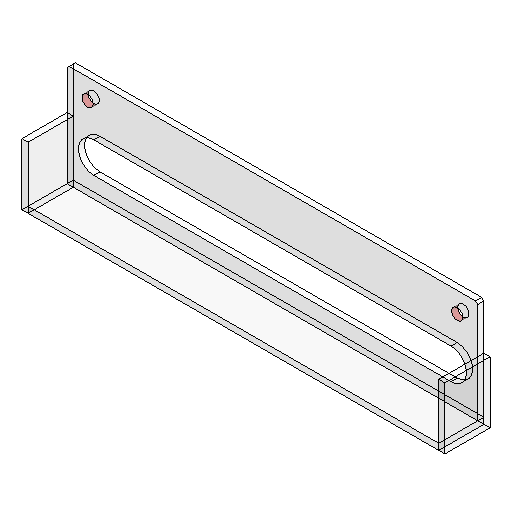
# Autodesk Inventor part: TL20240901-10320CV-027
Saved by Autodesk Inventor 2022.5 (Build 265521000, 521)
## iProperties
Category: FOLLOWER UNIT ASSY
Company: 현대 트랜시스
RuleStatus: InUse
Part Number: TL20240901-10320CV-027
Project: MEa-PJT 2LINE
Checked By: 김형민
Engr Approved By: 김형민
User Status: 2 x6
Material: PC
Description: 0
Document SubType Name: Modeling
Mfg Approved By: 호상태
Designer: USER106
Stock Number: 027
Density: 0.357273 g/cm^3
Appearance: Transparency
Detail Description: Processed products
Title: COVER
Subject: MEa차종 시트조립2라인
Author: USER106
Revision Number: A
Autodesk Inventor part; units mm, degrees
ref_plane "YZ Plane" through (0, 0, 0) normal (1, 0, 0) x (0, 1, 0)
ref_plane "XZ Plane" through (0, 0, 0) normal (0, 1, 0) x (-1, 0, 0)
ref_plane "XY Plane" through (0, 0, 0) normal (0, 0, 1) x (1, 0, 0)
sketch "Sketch2" plane through (0, 0, 0) normal (0, 1, 0) x (-1, 0, 0)
  line L0 (-100, -25) -> (100, -25)
  line L1 (100, -25) -> (100, 25)
  line L2 (100, 25) -> (-100, 25)
  line L3 (-100, 25) -> (-100, -25)
  line L4 (-100, -25) -> (100, 25) construction
  line L5 (100, -25) -> (-100, 25) construction
  point P0 (0, 0)
  dimension "d1" = 200
  dimension "d2" = 50
  constraints: 12 end point, 2 midpoint, 2 parallel, 1 horizontal, 1 perpendicular
  measures "d1" distance of L1.end L2.end
  measures "d2" distance of L0.end L1.end
extrude "Extrusion1" add sketch "Sketch2" along normal mid plane 3
sketch "Sketch3" plane through (100, -1.5, -25) normal (1, 0, 0) x (0, 0, -1)
  line L0 (-27, 3) -> (3, 3)
  line L1 (3, 3) -> (3, -19)
  line L2 (3, -19) -> (-27, -19)
  line L3 (-27, -19) -> (-27, 3)
  line L4 (0, 0) -> (0, 3) projected
  line L5 (-50, 3) -> (0, 3) projected
  point P0 (-25, 1.5)
  dimension "d13" = 3
  dimension "d14" = 22
  dimension "d15" = 30
  constraints: 8 end point, 2 parallel, 1 horizontal, 1 perpendicular, 1 point on line
  measures "d13" distance between parallel lines of L4 L1
  measures "d14" distance of L0.end L1.end
  measures "d15" distance of L0.start L0.end
extrude "Extrusion2" add sketch "Sketch3" along normal blind 3 separate body
extrude "Extrusion3" add sketch "Sketch3" against normal blind 3 from surface at -200 separate body
sketch "Sketch5" plane through (100, 1.5, -25) normal (0, 0, -1) x (-1, 0, 0)
  line L0 (200, -3) -> (200, 0) projected
  line L1 (200, 0) -> (0, 0)
  line L2 (0, 0) -> (0, -22)
  line L3 (0, -22) -> (200, -22)
  line L4 (200, -22) -> (200, 0)
  line L5 (0, -22) -> (0, 0) projected
  line L6 (0, -22) -> (-3, -22) projected
  point P0 (100, -1.5)
  constraints: 8 end point, 2 parallel, 2 point on line, 1 horizontal, 1 perpendicular
extrude "Extrusion5" add sketch "Sketch5" along normal blind 3 separate body
sketch "Sketch6" plane through (0, 1.5, 0) normal (0, 1, 0) x (1, 0, 0)
  line L0 (87, 7.5) -> (-87, 7.5) construction
  line L1 (87, 15) -> (-87, 15)
  line L2 (-87, 0) -> (87, 0)
  arc A0 (87, 0) -> (87, 15) centre (87, 7.5) ccw
  arc A1 (-87, 15) -> (-87, 0) centre (-87, 7.5) ccw
  line L3 (-100, -25) -> (100, -25) projected
  line L4 (-100, 28) -> (-100, -2) projected
  line L5 (100, 28) -> (100, -2) projected
  point P0 (0, 0)
  point P1 (0, 7.5)
  dimension "d40" = 32.5
  dimension "d41" = 13
  dimension "d43" = 13
  dimension "d44" = 15
  constraints: 8 end point, 4 point on circle, 4 tangent, 2 centre point, 1 horizontal, 1 midpoint, 1 parallel
  measures "d40" distance between parallel lines of L0 L3
  measures "d41" distance from line of L4 L0.end
  measures "d43" distance from line of L0.start L5
  measures "d44" distance between parallel lines of L2 L1
extrude "Extrusion6" cut sketch "Sketch6" along normal through all both and the other way through all bodies 1
sketch "Sketch7" plane through (0, 1.5, 0) normal (0, 1, 0) x (1, 0, 0)
  line L0 (-100, -25) -> (100, -25) projected
  line L1 (-100, 25) -> (-100, -25) projected
  line L2 (100, -25) -> (100, 25) projected
  point P0 (0, 0)
  point P1 (90, -15)
  point P2 (-90, -15)
  dimension "d34" = 10
  dimension "d35" = 10
  dimension "d36" = 10
  constraints: 1 horizontal alignment
  measures "d34" distance from line of point (-90, -15) L0
  measures "d35" distance from line of point (-90, -15) L1
  measures "d36" distance from line of point (90, -15) L2
hole "Hole1" at (90, 1.5, 15) at (-90, 1.5, 15) direction (0, -1, 0) diameter 5.5 end through all bodies 1 clearance for "Socket Head Cap Screw" size "M5" standard "TS Profile"
chamfer "Chamfer1" distance 1 angle 45 2 edges at (-100, 0, 25) (100, 0, 25)
equation "\"d36\" = d35"
body "Solid1"
body "Solid2"
body "Solid3"
body "Solid5"
